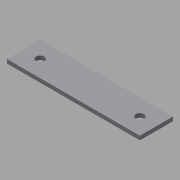
# Autodesk Inventor part: End Arm
Saved by Autodesk Inventor 2013 (Build 170138000, 138)
## iProperties
Created: 2013-02-08
Part Number: End Arm
Material: Generic
Document SubType Name: Modeling
Designer: Naphat
Density: 1 g/cm^3
Author: Naphat
Autodesk Inventor part; units mm, degrees
ref_plane "YZ Plane" through (0, 0, 0) normal (1, 0, 0) x (0, 1, 0)
ref_plane "XZ Plane" through (0, 0, 0) normal (0, 1, 0) x (-1, 0, 0)
ref_plane "XY Plane" through (0, 0, 0) normal (0, 0, 1) x (1, 0, 0)
sketch "Sketch1" plane through (0, 0, 0) normal (0, 1, 0) x (-1, 0, 0)
  line L0 (0, 0) -> (0, 25.4)
  line L1 (0, 25.4) -> (101.6, 25.4)
  line L2 (101.6, 25.4) -> (101.6, 0)
  line L3 (101.6, 0) -> (0, 0)
  dimension "d0" = 25.4
  dimension "d1" = 101.6
  constraints: 8 end point, 2 perpendicular, 1 parallel, 1 vertical
  measures "d0" distance of L0.start L0.end
  measures "d1" distance of L0.end L1.end
extrude "Extrusion1" add sketch "Sketch1" along normal blind 3
sketch "Sketch2" plane through (0, 3, 0) normal (0, 1, 0) x (1, 0, 0)
  line L0 (0, -25.4) -> (0, 0) projected
  line L1 (0, 0) -> (-101.6, 0) projected
  line L2 (-101.6, 0) -> (-101.6, -25.4) projected
  line L3 (-101.6, -25.4) -> (0, -25.4) projected
  line L4 (-101.6, 0) -> (-88.9, 0) construction
  line L5 (-88.9, 0) -> (-88.9, -25.4) construction
  line L6 (-101.6, 0) -> (-101.6, -12.7) construction
  line L7 (-101.6, -12.7) -> (0, -12.7) construction
  line L8 (0, 0) -> (-12.7, 0) construction
  line L9 (-12.7, 0) -> (-12.7, -25.4) construction
  circle A0 centre (-88.9, -12.7) radius 3.175
  circle A1 centre (-12.7, -12.7) radius 3.175
  dimension "d4" = 12.7
  dimension "d5" = 12.7
  dimension "d6" = 12.7
  dimension "d7" = 6.35
  dimension "d8" = 6.35
  constraints: 12 end point, 5 point on line, 4 midpoint, 2 centre point, 2 perpendicular
  measures "d4" distance of L1.end L4.end
  measures "d5" distance of L1.end L6.end
  measures "d6" distance of L0.end L8.end
  measures "d7" diameter of A0
  measures "d8" diameter of A1
hole "Hole1" at (-88.9, 3, 12.7) at (-12.7, 3, 12.7) direction (0, -1, 0) diameter 6.35 depth 25.4 tip angle 118
equation "\"d6\" = d4"
equation "\"d8\" = d7"
body "Solid1"
